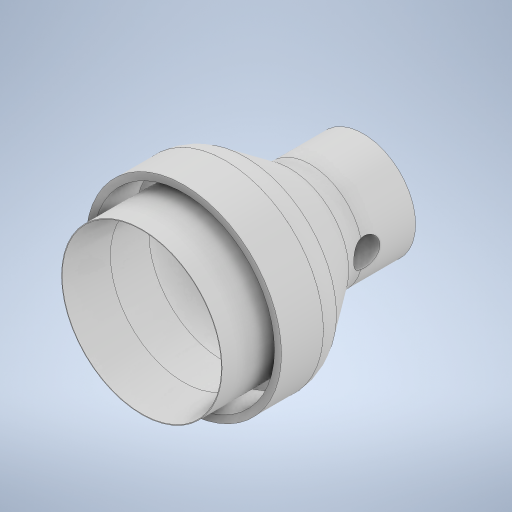
# Autodesk Inventor part: fly_funnel
Saved by Autodesk Inventor 2023.1 (Build 271208000, 208)
## iProperties
Created: 2022-12-15
Part Number: fly_funnel
Material: Generic
Document SubType Name: Modeling
Designer: dinesh
Density: 1 g/cm^3
Appearance: Default
Author: dinesh
Autodesk Inventor part; units mm, degrees
ref_plane "YZ Plane" through (0, 0, 0) normal (1, 0, 0) x (0, 1, 0)
ref_plane "XZ Plane" through (0, 0, 0) normal (0, 1, 0) x (-1, 0, 0)
ref_plane "XY Plane" through (0, 0, 0) normal (0, 0, 1) x (1, 0, 0)
sketch "Sketch1" plane through (0, 0, 0) normal (0, 1, 0) x (-1, 0, 0)
  line L0 (0, -27.5114) -> (0, 22.3977)
  line L1 (11.5, -6) -> (10.5, -6)
  line L2 (10.5, -6) -> (10.5, 0)
  line L3 (10.5, 0) -> (11.5, 0)
  line L4 (11.5, 0) -> (11.5, -6)
  line L5 (14, -7.5) -> (10.5, -7.5)
  line L6 (10.5, -5.5121) -> (10.5, -6)
  line L7 (10.5, -6) -> (14, -6)
  line L8 (14, -6) -> (14, -5.8832)
  line L9 (28.1307, 0) -> (-27.0173, 0)
  line L10 (7.5, -25.7) -> (6.5, -25.7)
  line L11 (6.5, -25.7) -> (6.5, -20.7)
  line L12 (6.5, -20.7) -> (7.5, -20.7)
  line L13 (7.5, -20.7) -> (7.5, -25.7)
  line L14 (5, -26.7) -> (2, -26.7)
  line L15 (2, -26.7) -> (2, -20.7)
  line L16 (2, -20.7) -> (5, -20.7)
  line L17 (5, -20.7) -> (5, -26.7)
  line L18 (7.5, -20.7) -> (2, -20.7)
  line L19 (2, -20.7) -> (2, -18.4879)
  line L20 (2, -16.5) -> (7.5, -16.5)
  line L21 (7.5, -18.1168) -> (7.5, -20.7)
  line L22 (3.3649, -15.0548) -> (9.1351, -8.9452)
  line L23 (8.4466, -15.1893) -> (13.0534, -8.8107)
  arc A0 (8.4466, -15.1893) -> (7.5, -18.1168) centre (12.5, -18.1168) ccw
  arc A1 (13.0534, -8.8107) -> (14, -5.8832) centre (9, -5.8832) ccw
  arc A2 (9.1351, -8.9452) -> (10.5, -5.5121) centre (5.5, -5.5121) ccw
  arc A3 (3.3649, -15.0548) -> (2, -18.4879) centre (7, -18.4879) ccw
  line L24 (13, -6) -> (14, -6)
  line L25 (14, -6) -> (14, 0)
  line L26 (14, 0) -> (13, 0)
  line L27 (13, 0) -> (13, -6)
  line L28 (11.5, 0) -> (11.5, 6)
  line L29 (11.5, 6) -> (11.4, 6)
  line L30 (11.4, 6) -> (10.5, 0)
  point P0 (0, 0)
  point P1 (11.5, -6)
  point P2 (13.9986, -6)
  point P3 (10.5, -5.5121)
  dimension "d2" = 1
  dimension "d4" = 1.5
  dimension "d5" = 6
  dimension "d6" = 6.5
  dimension "d7" = 1.5
  dimension "d8" = 1
  dimension "d9" = 4.2
  dimension "d10" = 5
  dimension "d11" = 9
  dimension "d12" = 2
  dimension "d13" = 5
  dimension "d14" = 5
  dimension "d15" = 5
  dimension "d17" = 6
  dimension "d20" = 1
  dimension "d21" = 6
  dimension "d22" = 1.5
  dimension "d23" = 13
  dimension "d28" = 6
  dimension "d29" = 0.1
  constraints: 62 end point, 12 parallel, 11 point on line, 8 horizontal, 8 point on circle, 8 tangent, 7 perpendicular, 4 centre point, 4 collinear, 2 vertical, 1 equal radius
  measures "d2" distance between parallel lines of L2 L4
  measures "d4" distance between parallel lines of L7 L5
  measures "d5" distance between parallel lines of L3 L1
  measures "d6" distance from line of point (0, 0) L11
  measures "d7" distance between parallel lines of L17 L11
  measures "d8" distance between parallel lines of L11 L13
  measures "d9" distance between parallel lines of L18 L20
  measures "d10" distance between parallel lines of L12 L10
  measures "d11" distance between parallel lines of L20 L5
  measures "d12" distance from line of point (0, 0) L15
  measures "d13" radius of A0
  measures "d14" radius of A1
  measures "d15" radius of A2
  measures "d17" distance between parallel lines of L16 L14
  measures "d20" distance between parallel lines of L27 L25
  measures "d21" distance between parallel lines of L7 L26
  measures "d22" distance between parallel lines of L27 L4
  measures "d23" distance from line of point (0, 0) L27
  measures "d28" distance of L3.end L28.end
  measures "d29" distance of L28.end L29.end
revolve "Revolution1" add sketch "Sketch1" angle 360 about axis through (0, 0, -27.5114) along (0, 0, 1) contours L7 A1 L23 A0 L21 L12 L18 L16 L19 A3 L22 A2 L2 L1 | L1 L2 L3 L4 | L3 L30 L29 L28 | L27 L9 L25 L8 L7 | L16 L17 L14 L15 | L13 L10 L11 L12
sketch "Sketch2" plane through (0, 0, 0) normal (1, 0, 0) x (0, 1, 0)
  line L0 (5, -26.7) -> (-5, -26.7) construction
  line L1 (0, -26.7) -> (0, -18.4879)
  line L2 (2, -18.4879) -> (-2, -18.4879) construction
  line L3 (5, -20.7) -> (-5, -20.7) construction
  circle A0 centre (0, -18.6) radius 2
  point P0 (0, 0)
  dimension "d18" = 4
  dimension "d19" = 2.1
  constraints: 2 end point, 2 midpoint, 1 centre point, 1 point on line
  measures "d18" diameter of A0
  measures "d19" distance from line of L3 A0.centre
extrude "Extrusion1" cut sketch "Sketch2" along normal blind 14 and the other way blind 2.5
equation "\"d18\" = ft_D"
equation "\"d19\" = 0.5 * ft_D + tol"
equation "\"d24\" = sv_OD + hw_thickness"
equation "\"d26\" = 0.5 * hw_thickness + 0.5 * ft_D"
equation "\"d2\" = hw_thickness"
equation "\"d4\" = 0.25 * hw_length"
equation "\"d5\" = hw_length"
equation "\"d6\" = 0.5 * sv_OD"
equation "\"d7\" = sv_thickness"
equation "\"d8\" = hw_thickness"
equation "\"d9\" = 1.05 * ft_D"
equation "\"d10\" = 0.833333 * hw_length"
equation "\"d11\" = 1.5 * hw_length"
equation "\"d12\" = 0.5 * ft_D"
equation "\"d13\" = fillet_D"
equation "\"d14\" = fillet_D"
equation "\"d15\" = fillet_D"
equation "\"d17\" = hw_length"
equation "\"d20\" = hw_thickness"
equation "\"d21\" = hw_length"
equation "\"d22\" = lv_thickness"
equation "\"d23\" = 0.5 * lv_OD"
equation "\"d28\" = hw_length"
equation "\"d29\" = tol"
equation "\"lv_OD\" = 26"
equation "\"lv_thickness\" = 1.5"
equation "\"hw_thickness\" = 1"
equation "\"hw_length\" = 6"
equation "\"sv_OD\" = 13"
equation "\"sv_thickness\" = 1.5"
equation "\"ft_D\" = 4"
equation "\"fillet_D\" = 5"
equation "\"tol\" = 0.1"
body "Solid1"
